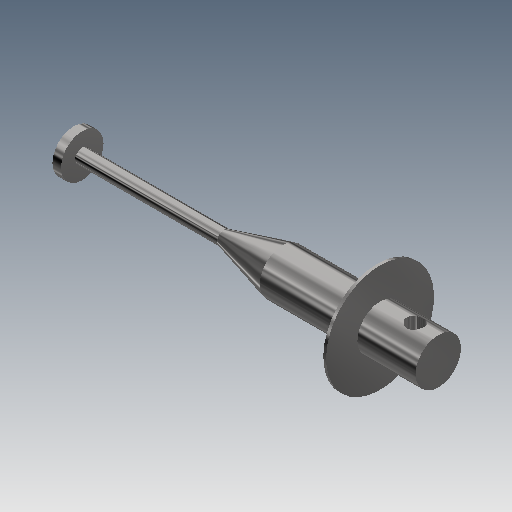
# Autodesk Inventor part: JF_0837B_Linear solenoid Pull 15N 12v1A Planger
Saved by Autodesk Inventor 2018.3 (Build 223284000, 284)
## iProperties
Manager: GURSKY
Company: ООО "МРФ-Инжиниринг"
Created: 2017-09-28
Part Number: JF_0837B_Linear solenoid Pull 15N 12v1A Planger
Project: 1708
Material: Сталь, нержавеющая, аустенитная
Catalog Web Link: http://mrfengineering.com.ua/
Vendor: ltd "MRF-ENGINEERING"
Document SubType Name: Modeling
Designer: Макс
Engineer: TIHONOV
Authority: GURSKY
Stock Number: 1708
Density: 8 g/cm^3
Appearance: Нержавеющая — полированная
Title: ---
Subject: Filling mashine
Author: Макс
Autodesk Inventor part; units mm, degrees
ref_plane "YZ Plane" through (0, 0, 0) normal (1, 0, 0) x (0, 1, 0)
ref_plane "XZ Plane" through (0, 0, 0) normal (0, 1, 0) x (-1, 0, 0)
ref_plane "XY Plane" through (0, 0, 0) normal (0, 0, 1) x (1, 0, 0)
sketch "Эскиз1" plane through (0, 0, 0) normal (0, 0, 1) x (1, 0, 0)
  line L0 (0, 0) -> (0, 7.5)
  line L1 (0, 7.5) -> (3, 7.5)
  line L2 (3, 7.5) -> (3, 2.5)
  line L3 (3, 2.5) -> (53, 2.5)
  line L4 (53, 2.5) -> (73.5263, 8)
  line L5 (128.4, 8) -> (128.4, 0)
  line L6 (128.4, 0) -> (0, 0)
  line L7 (107.9, 8) -> (107.9, 19)
  line L8 (107.9, 19) -> (106.9, 19)
  line L9 (106.9, 19) -> (106.9, 8)
  line L10 (73.5263, 8) -> (106.9, 8)
  line L11 (107.9, 8) -> (128.4, 8)
  dimension "d0" = 5
  dimension "d1" = 15
  dimension "d2" = 3
  dimension "d3" = 128.4
  dimension "d4" = 15
  dimension "d6" = 50
  dimension "d12" = 1
  dimension "d13" = 16
  dimension "d14" = 21.5
  dimension "d15" = 38
  constraints: 24 end point, 4 perpendicular, 2 horizontal, 1 coincident, 1 collinear, 1 parallel, 1 vertical
  measures "d0" diameter of L3 L6
  measures "d1" diameter of L1 L6
  measures "d2" distance of L0.end L1.end
  measures "d3" distance between parallel lines of L5 L0
  measures "d4" angle of L4 L3
  measures "d6" distance of L2.end L3.end
  measures "d12" distance of L8.end L7.end
  measures "d13" diameter of L10 L6
  measures "d14" distance between parallel lines of L5 L9
  measures "d15" diameter of L8 L6
revolve "Вращение1" add sketch "Эскиз1" angle 360 about axis through (128.4, 0, 0) along (-1, 0, 0)
sketch "Эскиз2" plane through (0, 0, 0) normal (0, 1, 0) x (-1, 0, 0)
  circle A0 centre (-120.4, 0) radius 3
  line L0 (-128.4, 8) -> (-128.4, -8) projected
  point P0 (0, 0)
  point P1 (-128.4, 0)
  dimension "d8" = 6
  dimension "d9" = 8
  constraints: 1 centre point, 1 horizontal alignment, 1 midpoint
  measures "d8" diameter of A0
  measures "d9" distance from line of L0 A0.centre
extrude "Выдавливание1" cut sketch "Эскиз2" along normal through all both and the other way through all
